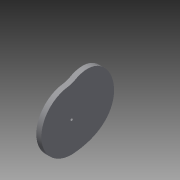
# Autodesk Inventor part: plateCamPart
Saved by Autodesk Inventor 2015 (Build 190159000, 159)
## iProperties
Created: 2015-04-14
Part Number: plateCamPart
Material: Generic
Document SubType Name: Modeling
Designer: WASHHSST
Density: 1 g/cm^3
Appearance: Default
Author: WASHHSST
Autodesk Inventor part; units mm, degrees
ref_plane "YZ Plane" through (0, 0, 0) normal (1, 0, 0) x (0, 1, 0)
ref_plane "XZ Plane" through (0, 0, 0) normal (0, 1, 0) x (-1, 0, 0)
ref_plane "XY Plane" through (0, 0, 0) normal (0, 0, 1) x (1, 0, 0)
sketch "Sketch1" plane through (0, 0, 0) normal (1, 0, 0) x (0, 1, 0)
  circle A0 centre (0, 0) radius 76.2
  spline S0 degree 3 poles (76.2, 0) (145.5168, -95.878) (-64.2426, -180.0292) (-76.2, 0) knots 0 0 0 0 1 1 1 1
  point P0 (76.2, -76.2)
  point P1 (0, -105.0953)
  dimension "d0" = 152.4
  constraints: 2 point on circle, 1 centre point, 1 coincident, 4 other
  measures "d0" diameter of A0
extrude "Extrusion1" add sketch "Sketch1" along normal blind 12.7
fillet "Fillet1" radius 50.8 1 edges at (6.35, 76.2, 0)
sketch "Sketch2" plane through (12.7, 0, 0) normal (1, 0, 0) x (0, 0, -1)
  arc A0 (-9.8256, 75.5639) -> (0, -76.2) centre (0, 0) ccw projected
  constraints: 1 coincident
hole "Hole1" at (12.7, 0, 0) direction (-1, 0, 0) diameter 6.35 end through all
body "Solid1"
